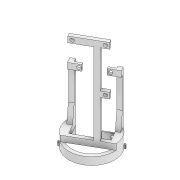
# Autodesk Inventor part: Sujeccion_PCBs
Saved by Autodesk Inventor 2022.3 (Build 263350000, 350)
## iProperties
Created: 2023-07-18
Part Number: Sujeccion_PCBs
Material: Genérico
Document SubType Name: Modeling
Designer: Usuario
Density: 1 g/cm^3
Appearance: Valor por defecto
Author: Usuario
Autodesk Inventor part; units mm, degrees
ref_plane "YZ Plane" through (0, 0, 0) normal (1, 0, 0) x (0, 1, 0)
ref_plane "XZ Plane" through (0, 0, 0) normal (0, 1, 0) x (-1, 0, 0)
ref_plane "XY Plane" through (0, 0, 0) normal (0, 0, 1) x (1, 0, 0)
sketch "Boceto1" plane through (0, 0, 0) normal (0, 1, 0) x (-1, 0, 0)
  arc A0 (-14.0673, -14.2166) -> (-10.4918, -17.0271) centre (0, 0) ccw
  line L0 (1.1244, -10.3205) -> (-10.4918, -17.0271)
  line L1 (1.6244, -11.1865) -> (1.1244, -10.3205)
  line L2 (19.9915, -0.5822) -> (1.6244, -11.1865)
  arc A1 (19.9915, -0.5822) -> (19.8537, 2.4146) centre (0, 0) ccw
  line L3 (20.8464, 2.5353) -> (19.8537, 2.4146)
  arc A2 (20.8464, 2.5353) -> (15.7326, 13.9099) centre (0, 0) ccw
  line L4 (15.7326, 13.9099) -> (14.6319, 13.6347)
  arc A3 (14.6319, 13.6347) -> (-19.8205, -2.6736) centre (0, 0) ccw
  line L5 (-20.7178, -3.431) -> (-19.8205, -2.6736)
  arc A4 (-20.7178, -3.431) -> (-14.9337, -14.7643) centre (0, 0) ccw
  line L6 (-14.9337, -14.7643) -> (-14.0673, -14.2166)
  line L7 (19.1288, 5.8387) -> (20.1107, 6.0466)
  arc A5 (20.1107, 6.0466) -> (-20.7178, -3.431) centre (0, 0) ccw
  line L8 (-20.7178, -3.431) -> (-19.8205, -2.6736)
  arc A6 (19.1288, 5.8387) -> (-19.8205, -2.6736) centre (0, 0) ccw
  line L9 (20.8464, 2.5353) -> (19.8537, 2.4146)
  arc A7 (19.9915, -0.5822) -> (19.8537, 2.4146) centre (0, 0) ccw
  line L10 (19.9915, -0.5822) -> (21, 0)
  arc A8 (21, 0) -> (20.8464, 2.5353) centre (0, 0) ccw
  line L11 (-18.8764, -6.6092) -> (-19.6914, -7.2971)
  arc A9 (-19.6914, -7.2971) -> (-10.5, -18.1865) centre (0, 0) ccw
  line L12 (-10.5, -18.1865) -> (1.6244, -11.1865)
  line L13 (1.6244, -11.1865) -> (1.1244, -10.3205)
  line L14 (1.1244, -10.3205) -> (-10.4918, -17.0271)
  arc A10 (-18.8764, -6.6092) -> (-10.4918, -17.0271) centre (0, 0) ccw
  circle A11 centre (0, 0) radius 19.75
  line L15 (1.1244, -10.3205) -> (0.9994, -10.104)
  line L16 (0.9994, -10.104) -> (-10.4871, -16.7357)
  line L17 (0.9994, -10.104) -> (19.7371, 0.7142)
  circle A12 centre (0, 0) radius 16.75
  line L18 (0.9994, -10.104) -> (0.4994, -9.238)
  line L19 (0.4994, -9.238) -> (-8.4018, -14.4904)
  point P0 (16.552, -2.5681)
  point P1 (19.7365, -0.7295)
  dimension "d2" = 33.5
  dimension "d0" = 39.5
  dimension "d1" = 0.25
  dimension "d3" = 1
  constraints: 40 end point, 24 point on circle, 12 centre point, 2 coincident, 2 perpendicular, 1 point on line, 3 other
  measures "d0" diameter of A11
  measures "d1" distance of L13.end L15.end
  measures "d3" distance of L15.end L18.end
extrude "Extrusión1" add sketch "Boceto1" along normal blind 6.5 contours A11 L17 A12 L16 | A12 L19 L18 L16 | A11 L2 A12 L17
sketch "Boceto2" plane through (0, 0, 0) normal (0, 1, 0) x (-1, 0, 0)
  arc A0 (14.6319, 13.6347) -> (-19.8205, -2.6736) centre (0, 0) ccw
  arc A1 (19.1288, 5.8387) -> (-19.8205, -2.6736) centre (0, 0) ccw
  arc A2 (20.1107, 6.0466) -> (-20.7178, -3.431) centre (0, 0) ccw
  line L0 (19.9915, -0.5822) -> (1.6244, -11.1865)
  line L1 (15.7326, 13.9099) -> (14.6319, 13.6347)
  arc A3 (19.9915, -0.5822) -> (19.8537, 2.4146) centre (0, 0) ccw
  arc A4 (19.9915, -0.5822) -> (19.8537, 2.4146) centre (0, 0) ccw
  line L2 (19.9915, -0.5822) -> (21, 0)
  arc A5 (21, 0) -> (20.8464, 2.5353) centre (0, 0) ccw
  line L3 (19.1288, 5.8387) -> (20.1107, 6.0466)
  line L4 (20.8464, 2.5353) -> (19.8537, 2.4146)
  line L5 (20.8464, 2.5353) -> (19.8537, 2.4146)
  arc A6 (20.8464, 2.5353) -> (15.7326, 13.9099) centre (0, 0) ccw
  line L6 (1.6244, -11.1865) -> (1.1244, -10.3205)
  arc A7 (-14.0673, -14.2166) -> (-10.4918, -17.0271) centre (0, 0) ccw
  line L7 (1.1244, -10.3205) -> (-10.4918, -17.0271)
  arc A8 (-20.7178, -3.431) -> (-14.9337, -14.7643) centre (0, 0) ccw
  line L8 (-14.9337, -14.7643) -> (-14.0673, -14.2166)
  line L9 (-18.8764, -6.6092) -> (-19.6914, -7.2971)
  line L10 (1.6244, -11.1865) -> (1.1244, -10.3205)
  arc A9 (-18.8764, -6.6092) -> (-10.4918, -17.0271) centre (0, 0) ccw
  arc A10 (-19.6914, -7.2971) -> (-10.5, -18.1865) centre (0, 0) ccw
  line L11 (1.1244, -10.3205) -> (-10.4918, -17.0271)
  line L12 (-10.5, -18.1865) -> (1.6244, -11.1865)
  line L13 (-20.7178, -3.431) -> (-19.8205, -2.6736)
  line L14 (-20.7178, -3.431) -> (-19.8205, -2.6736)
  circle A11 centre (0, 0) radius 19.75
  line L15 (1.1244, -10.3205) -> (0.9994, -10.104)
  line L16 (0.9994, -10.104) -> (-10.4871, -16.7357)
  line L17 (0.9994, -10.104) -> (19.7371, 0.7142)
  circle A12 centre (0, 0) radius 16.75
  line L18 (0.9994, -10.104) -> (0.4994, -9.238)
  line L19 (0.4994, -9.238) -> (-8.4018, -14.4904)
  line L20 (-14.9337, -14.7643) -> (-13.8504, -14.0794)
  arc A13 (19.7365, -0.7295) -> (-10.4871, -16.7357) centre (0, 0) ccw projected
  line L21 (-16.2705, -13.2767) -> (-15.2057, -12.6035)
  line L22 (14.6319, 13.6347) -> (14.3543, 13.5653)
  line L23 (16.9845, 12.3502) -> (15.8956, 11.7215)
  point P0 (16.552, -2.5681)
  dimension "d8" = 33.5
  dimension "d6" = 39.5
  dimension "d7" = 0.25
  dimension "d9" = 1
  dimension "d10" = 2
  dimension "d11" = 2
  constraints: 48 end point, 30 point on circle, 12 centre point, 2 coincident, 2 perpendicular, 2 point on line, 1 parallel, 3 other
  measures "d6" diameter of A11
  measures "d7" distance of L10.end L15.end
  measures "d9" distance of L15.end L18.end
  measures "d10" distance of L8.start L21.start
  measures "d11" distance of L1.start L23.start
extrude "Extrusión2" add sketch "Boceto2" along normal blind 2.4 contours L1 A2 L23 A1 | A1 L23 A11 L22 | A11 L20 A9 L21 | A9 L8 A8 L21
sketch "Boceto3" plane through (-0.9994, 0, -10.104) normal (-0.5, 0, -0.8660254) x (-0.8660254, 0, 0.5)
  line L0 (0, 0) -> (0, 6.5) projected
  line L1 (0, 3.25) -> (-7, 3.25)
  circle A0 centre (-7, 3.25) radius 1.5
  point P0 (4.1865, 0)
  dimension "d14" = 7
  dimension "d15" = 3
  constraints: 2 end point, 1 centre point, 1 coincident, 1 horizontal, 1 midpoint
  measures "d14" distance of L1.start L1.end
  measures "d15" diameter of A0
extrude "Extrusión3" cut sketch "Boceto3" against normal blind 1
sketch "Boceto5" plane through (0, 6.5, 0) normal (0, 1, 0) x (1, 0, 0)
  arc A0 (-19.7365, 0.7295) -> (10.4871, 16.7357) centre (0, 0) ccw projected
  circle A1 centre (0, 0) radius 19.75
  arc A2 (-16.552, 2.5681) -> (8.4018, 14.4904) centre (0, 0) ccw projected
  circle A3 centre (0, 0) radius 16.75
  line L0 (-16.552, 2.5681) -> (-19.7365, 0.7295) projected
  line L1 (-16.552, 2.5681) -> (-19.7365, 0.7295)
  line L2 (10.4871, 16.7357) -> (7.4684, 14.9929)
  line L3 (10.4871, 16.7357) -> (-0.9994, 10.104) projected
  line L4 (-0.9994, 10.104) -> (8.0006, -5.4845)
  line L5 (8.0006, -5.4845) -> (6.5006, -2.8864)
  line L6 (6.5006, -2.8864) -> (16.4994, 2.8864)
  line L7 (6.5006, -2.8864) -> (-10.7494, -12.8457)
  line L8 (7.4684, 14.9929) -> (14.9684, 2.0025)
  line L9 (-16.552, 2.5681) -> (-8.427, -11.5048)
  line L10 (8.0006, -5.4845) -> (19.7088, 1.2752)
  line L11 (8.0006, -5.4845) -> (-10.9588, -16.4307)
  point P0 (19.7088, 1.2752)
  point P1 (-10.9588, -16.4307)
  dimension "d18" = 18
  dimension "d22" = 3
  constraints: 20 end point, 7 point on circle, 6 point on line, 2 centre point, 2 coincident, 2 perpendicular, 1 collinear
  measures "d18" distance of L3.end L4.end
  measures "d22" distance of L4.end L5.end
extrude "Extrusión4" add sketch "Boceto5" along normal blind 5 contours L0 A2 L11 A0 | A0 L10 A2 A3 L2 | L9 L7 A2 | A2 L7 L4 L11 | A3 A2 L6 L8 | L10 L4 L6 A2
sketch "Boceto7" plane through (0, 11.5, 0) normal (0, 1, 0) x (1, 0, 0)
  line L0 (7.4684, 14.9929) -> (14.9684, 2.0025) projected
  line L1 (7.4684, 14.9929) -> (8.4684, 13.2608)
  arc A0 (19.7088, 1.2752) -> (10.4871, 16.7357) centre (0, 0) ccw projected
  line L2 (10.4871, 16.7357) -> (11.4871, 15.0036)
  line L3 (8.4684, 13.2608) -> (11.4871, 15.0036)
  line L4 (7.922, 14.2073) -> (14.9684, 2.0025) projected
  line L5 (-16.552, 2.5681) -> (-19.7365, 0.7295) projected
  line L6 (-16.552, 2.5681) -> (-14.927, -0.2465)
  line L7 (-8.427, -11.5048) -> (-16.552, 2.5681) projected
  line L8 (-19.7365, 0.7295) -> (-18.1115, -2.0851)
  line L9 (-18.1115, -2.0851) -> (-14.927, -0.2465)
  line L10 (10.4871, 16.7357) -> (7.4684, 14.9929)
  line L11 (10.4871, 16.7357) -> (-0.9994, 10.104) projected
  dimension "d23" = 2
  constraints: 14 end point, 3 point on line, 2 perpendicular, 1 collinear, 1 parallel
  measures "d23" distance of L0.start L1.end
extrude "Extrusión5" add sketch "Boceto7" along normal blind 45
chamfer "Chaflán1" distance 14 angle 15 1 edges at (9.9777, 11.5, -14.1322) measured on face at (9.4746, 26.5, -13.8418)
chamfer "Chaflán2" distance 14 angle 15 1 edges at (-16.5192, 11.5, 1.1658) measured on face at (-17.05, 26.5, 1.4722)
sketch "Boceto8" plane through (0, 56.5, 0) normal (0, 1, 0) x (1, 0, 0)
  line L0 (11.4871, 15.0036) -> (8.4684, 13.2608) projected
  line L1 (11.4871, 15.0036) -> (12.4871, 13.2716)
  line L2 (12.4871, 13.2716) -> (9.4684, 11.5288)
  line L3 (7.922, 14.2073) -> (14.9684, 2.0025) projected
  line L4 (9.4684, 11.5288) -> (8.4684, 13.2608)
  line L5 (8.4684, 13.2608) -> (11.4871, 15.0036)
  line L6 (12.4871, 13.2716) -> (4.6929, 8.7716)
  line L7 (4.6929, 8.7716) -> (3.6929, 10.5036)
  line L8 (3.6929, 10.5036) -> (8.4684, 13.2608)
  line L9 (-16.2359, -5.3338) -> (-19.7365, 0.7295) projected
  line L10 (-18.1115, -2.0851) -> (-17.1115, -3.8172)
  line L11 (-17.1115, -3.8172) -> (-9.3173, 0.6828)
  line L12 (-9.3173, 0.6828) -> (-10.3173, 2.4149)
  line L13 (-14.927, -0.2465) -> (-18.1115, -2.0851) projected
  line L14 (-10.3173, 2.4149) -> (-18.1115, -2.0851)
  point P0 (0, 0)
  dimension "d32" = 2
  dimension "d33" = 9
  dimension "d34" = 9
  constraints: 22 end point, 7 point on line, 6 perpendicular, 1 collinear, 1 parallel
  measures "d32" distance of L0.start L1.end
  measures "d33" distance of L1.end L6.end
  measures "d34" distance of L10.end L11.end
extrude "Extrusión6" add sketch "Boceto8" against normal blind 5
sketch "Boceto9" plane through (8.4684, 51.5, -13.2608) normal (-0.5, 0, -0.8660254) x (-0.8660254, 0, 0.5)
  line L0 (0, -45) -> (0, 5) projected
  line L1 (0, 5) -> (0, 0)
  line L2 (-3.4857, 0) -> (5.5143, 0) projected
  line L3 (0, 2.5) -> (27.0146, 2.5)
  line L4 (27.0146, -45) -> (27.0146, 5) projected
  line L5 (13.5073, 2.5) -> (3.5073, 2.5)
  line L6 (13.5073, 2.5) -> (23.5073, 2.5)
  circle A0 centre (3.5073, 2.5) radius 1.5
  circle A1 centre (23.5073, 2.5) radius 1.5
  point P0 (13.9642, -51.5)
  dimension "d37" = 10
  dimension "d38" = 10
  dimension "d39" = 3
  dimension "d40" = 3
  constraints: 8 end point, 4 point on line, 2 centre point, 2 coincident, 2 midpoint, 1 perpendicular, 1 vertical
  measures "d37" distance of L5.start L5.end
  measures "d38" distance of L5.start L6.end
  measures "d39" diameter of A0
  measures "d40" diameter of A1
extrude "Extrusión7" cut sketch "Boceto9" against normal through all
sketch "Boceto10" plane through (0, 11.5, 0) normal (0, 1, 0) x (1, 0, 0)
  line L0 (19.7088, 1.2752) -> (11.0485, -3.7248)
  line L1 (-7.9943, -14.7192) -> (16.7443, -0.4363) projected
  line L2 (11.0485, -3.7248) -> (9.5485, -1.1267)
  line L3 (9.5485, -1.1267) -> (6.0844, -3.1267)
  line L4 (14.9684, 2.0025) -> (-8.427, -11.5048) projected
  line L5 (6.0844, -3.1267) -> (7.5844, -5.7248)
  line L6 (7.5844, -5.7248) -> (11.0485, -3.7248)
  point P0 (0, 0)
  dimension "d43" = 10
  dimension "d44" = 4
  constraints: 10 end point, 3 perpendicular, 3 point on line
  measures "d43" distance of L0.start L0.end
  measures "d44" distance of L2.end L3.end
extrude "Extrusión8" add sketch "Boceto10" along normal blind 75
sketch "Boceto11" plane through (9.5485, 11.5, 1.1267) normal (0.8660254, 0, -0.5) x (-0.5, 0, -0.8660254)
  line L0 (-3, 75) -> (0, 75) projected
  line L1 (-3, 0) -> (-3, 75) projected
  line L2 (0, 75) -> (-3, 75)
  line L3 (-3, 75) -> (-3, 70)
  line L4 (-3, 70) -> (0, 70)
  line L5 (0, 70) -> (0, 75)
  point P0 (5.75, -11.5)
  dimension "d47" = 5
  constraints: 8 end point, 2 parallel, 1 horizontal, 1 perpendicular, 1 point on line
  measures "d47" distance of L3.end L2.end
extrude "Extrusión9" add sketch "Boceto11" along normal blind 6
sketch "Boceto12" plane through (7.5844, 11.5, 5.7248) normal (-0.8660254, 0, 0.5) x (0.5, 0, 0.8660254)
  line L0 (-3, 75) -> (0, 75) projected
  line L1 (0, 75) -> (0, 70) projected
  line L2 (0, 70) -> (-3, 70) projected
  line L3 (-3, 70) -> (-3, 75) projected
  point P0 (-8.75, -11.5)
extrude "Extrusión10" add sketch "Boceto12" along normal blind 16.5
sketch "Boceto13" plane through (19.7088, 6.5, -1.2752) normal (0.5, 0, 0.8660254) x (0.8660254, 0, -0.5)
  line L0 (-30.5, 80) -> (-30.5, 75) projected
  line L1 (-30.5, 77.5) -> (-4, 77.5)
  line L2 (-4, 80) -> (-4, 75) projected
  line L3 (-17.25, 77.5) -> (-27.75, 77.5)
  line L4 (-17.25, 77.5) -> (-6.75, 77.5)
  circle A0 centre (-27.75, 77.5) radius 1.5
  circle A1 centre (-6.75, 77.5) radius 1.5
  point P0 (-17.7059, -6.5)
  dimension "d52" = 10.5
  dimension "d53" = 10.5
  dimension "d54" = 3
  dimension "d55" = 3
  constraints: 6 end point, 3 midpoint, 2 centre point, 2 coincident, 2 point on line
  measures "d52" distance of L3.start L3.end
  measures "d53" distance of L3.start L4.end
  measures "d54" diameter of A0
  measures "d55" diameter of A1
extrude "Extrusión11" cut sketch "Boceto13" against normal through all
sketch "Boceto14" plane through (19.7088, 6.5, -1.2752) normal (0.5, 0, 0.8660254) x (0.8660254, 0, -0.5)
  line L0 (-10, 5) -> (-10, 75) projected
  line L1 (-10, 75) -> (-10, 42.7)
  line L2 (-10, 42.7) -> (-4, 42.7)
  line L3 (-3.7417, 0) -> (-3.7417, 50) projected
  line L4 (-4, 42.7) -> (-4, 37.7)
  line L5 (-4, 42.7) -> (1, 42.7) construction
  line L6 (-4, 37.7) -> (-10, 37.7)
  line L7 (-10, 37.7) -> (-10, 42.7)
  circle A0 centre (-6.75, 77.5) radius 1.5 projected
  line L8 (-6.75, 77.5) -> (-6.75, 40.2)
  circle A1 centre (-6.75, 40.2) radius 1.5
  point P0 (-17.7059, -6.5)
  dimension "d58" = 32.3
  dimension "d59" = 6
  dimension "d60" = 5
  dimension "d61" = 90
  dimension "d65" = 37.3
  dimension "d66" = 3
  constraints: 14 end point, 3 perpendicular, 2 point on line, 1 centre point, 1 coincident, 1 collinear, 1 horizontal, 1 vertical
  measures "d58" distance of L0.end L1.end
  measures "d59" distance of L1.end L2.end
  measures "d60" distance of L2.end L4.end
  measures "d61" angle of L4 L5
  measures "d65" distance of L8.start L8.end
  measures "d66" diameter of A1
extrude "Extrusión12" add sketch "Boceto14" against normal blind 3 contours L0 L2 L4 L6
